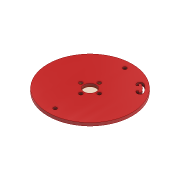
# Autodesk Inventor part: 615468 outer plate
Saved by Autodesk Inventor 2020 (Build 240168000, 168)
## iProperties
Created: 2017-11-20
Part Number: 615468 outer plate
Material: Generic
Document SubType Name: Modeling
Designer: ball
Density: 1 g/cm^3
Appearance: Default
Author: ball
Revision Number: ANY
Autodesk Inventor part; units mm, degrees
ref_plane "YZ Plane" through (0, 0, 0) normal (1, 0, 0) x (0, 1, 0)
ref_plane "XZ Plane" through (0, 0, 0) normal (0, 1, 0) x (-1, 0, 0)
ref_plane "XY Plane" through (0, 0, 0) normal (0, 0, 1) x (1, 0, 0)
ref_plane "Work Plane1" through (0, 1.5875, 0) normal (0, 1, 0) x (1, 0, 0)
sketch "Sketch1" plane through (0, 1.5875, 0) normal (0, 1, 0) x (1, 0, 0)
  circle A0 centre (0, 0) radius 44.45
  circle A1 centre (0, -9.779) radius 1.778 construction
  circle A2 centre (-9.779, 0) radius 1.778 construction
  circle A3 centre (0, 9.779) radius 1.778 construction
  circle A4 centre (9.779, 0) radius 1.778 construction
  circle A5 centre (0, 0) radius 6.35 construction
  circle A6 centre (0, -9.779) radius 1.9304
  circle A7 centre (-9.779, 0) radius 1.9304
  circle A8 centre (0, 9.779) radius 1.9304
  circle A9 centre (9.779, 0) radius 1.9304
  circle A10 centre (0, 0) radius 6.477
  circle A11 centre (0, 0) radius 34.925 construction
  circle A12 centre (0, -36.83) radius 1.9304
  circle A13 centre (0, 36.83) radius 1.9304
  line L0 (0, 0) -> (31.4309, 31.4309) construction
  line L1 (0, 0) -> (44.45, 0) construction
  line L2 (28.8087, 22.5367) -> (28.1119, 23.6217)
  line L3 (22.1752, 26.6653) -> (23.6324, 28.1226)
  line L4 (23.6324, 28.1226) -> (22.5367, 28.8087)
  line L5 (21.5127, 27.0801) -> (22.1752, 26.6653)
  line L6 (28.1119, 23.6217) -> (26.6653, 22.1752)
  arc A14 (28.8087, 22.5367) -> (30.8149, 23.7252) centre (29.8118, 23.131) ccw
  arc A15 (23.7252, 30.8149) -> (22.5367, 28.8087) centre (23.131, 29.8118) ccw
  arc A16 (24.7492, 32.5435) -> (21.5127, 27.0801) centre (23.131, 29.8118) ccw
  arc A17 (27.0801, 21.5127) -> (32.5435, 24.7492) centre (29.8118, 23.131) ccw
  arc A18 (30.8149, 23.7252) -> (23.7252, 30.8149) centre (13.4217, 13.4217) ccw
  arc A19 (32.5435, 24.7492) -> (24.7492, 32.5435) centre (13.4217, 13.4217) ccw
  line L7 (27.0801, 21.5127) -> (26.6653, 22.1752)
  point P0 (24.7492, 32.5435)
  dimension "d1" = 88.9
  dimension "d2" = 3.8608
  dimension "d3" = 3.8608
  dimension "d5" = 3.8608
  dimension "d6" = 12.954
  dimension "d7" = 69.85
  dimension "d8" = 3.8608
  dimension "d10" = 3.8608
  dimension "d11" = 36.83
  dimension "d12" = 45
  dimension "d13" = 36.83
  constraints: 16 end point, 14 centre point, 12 point on circle, 10 coincident, 1 equal length, 1 horizontal, 1 parallel, 1 point on line, 3 other
  measures "d2" diameter of A6
  measures "d3" diameter of A7
  measures "d5" diameter of A9
  measures "d6" diameter of A10
  measures "d7" diameter of A11
  measures "d8" diameter of A12
  measures "d10" diameter of A13
  measures "d11" distance of point (0, 0) A13.centre
  measures "d12" angle of L1 L0
  measures "d13" distance of point (0, 0) A12.centre
extrude "Extrusion1" add sketch "Sketch1" along normal mid plane 3.175
body "Solid2"
